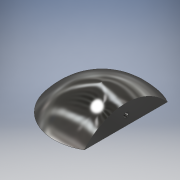
# Autodesk Inventor part: camera side 2
Saved by Autodesk Inventor 2017 (Build 210142000, 142)
## iProperties
Created: 2020-02-20
Part Number: camera side 2
Material: Silicon Nitride
Document SubType Name: Modeling
Designer: S346852600
Density: 3.18 g/cm^3
Appearance: Chrome - Polished Black
Author: S346852600
Autodesk Inventor part; units mm, degrees
ref_plane "YZ Plane" through (0, 0, 0) normal (1, 0, 0) x (0, 1, 0)
ref_plane "XZ Plane" through (0, 0, 0) normal (0, 1, 0) x (-1, 0, 0)
ref_plane "XY Plane" through (0, 0, 0) normal (0, 0, 1) x (1, 0, 0)
sketch "Sketch1" plane through (0, 0, 0) normal (1, 0, 0) x (0, 1, 0)
  line L0 (0, 0) -> (0, 25.4)
  line L1 (0, 0) -> (13.97, 0)
  arc A0 (13.97, 0) -> (0, 25.4) centre (-21.4675, -2.9489) ccw
  line L2 (0, 0) -> (0, 15.748)
  line L3 (0, 15.748) -> (8.7805, 15.748)
  dimension "d0" = 25.4
  dimension "d1" = 13.97
  dimension "d2" = 35.56
  dimension "d3" = 15.748
  constraints: 8 end point, 3 point on circle, 1 centre point, 1 horizontal, 1 perpendicular, 1 point on line, 1 vertical
  measures "d0" distance of L0.start L0.end
  measures "d1" distance of L0.start L1.end
  measures "d2" radius of A0
  measures "d3" distance of L0.start L2.end
revolve "Revolution1" add sketch "Sketch1" angle 360 about axis through (0, 0, 0) along (0, 1, 0)
sketch "Sketch6" plane through (0, 0, 0) normal (0, -1, 0) x (0, 0, -1)
  circle A0 centre (0, 0) radius 1.27
  dimension "d19" = 2.54
  constraints: 1 centre point, 1 coincident
  measures "d19" diameter of A0
extrude "Extrusion5" cut sketch "Sketch6" against normal blind 2.54
sketch "Sketch7" plane through (0, 0, 0) normal (0, -1, 0) x (0, 0, -1)
  point P0 (0, 0)
sketch "Sketch8" plane through (0, 0, 0) normal (0, -1, 0) x (1, 0, 0)
  circle A0 centre (0, 0) radius 1.27 projected
  line L0 (0, 0) -> (12.657, 0)
  line L1 (12.657, 0) -> (12.657, 22.0218)
  circle A1 centre (0, 0) radius 25.4 projected
  line L2 (12.657, 22.0218) -> (27.5297, 22.0218)
  line L3 (27.5297, 22.0218) -> (27.5297, -29.4448)
  line L4 (27.5297, -29.4448) -> (12.657, -29.4448)
  line L5 (12.657, -29.4448) -> (12.657, 22.0218)
  dimension "d22" = 22.0218
  constraints: 12 end point, 2 horizontal, 2 parallel, 2 perpendicular, 2 other
  measures "d22" distance of L0.end L1.end
extrude "Extrusion6" cut sketch "Sketch8" against normal blind 25.4 contours L1 A1 L5 | L2 L3 L4 L5 A1 picked at (14.0935, 13.6414)
sketch "Sketch9" plane through (12.657, 0, 22.0218) normal (1, 0, 0) x (0, 0, -1)
  line L0 (22.0218, 0) -> (22.0218, 5.08)
  circle A0 centre (22.0218, 5.08) radius 1.27
  dimension "d25" = 5.08
  dimension "d26" = 2.54
  constraints: 2 end point, 1 centre point, 1 coincident, 1 vertical
  measures "d25" distance of L0.start L0.end
  measures "d26" diameter of A0
extrude "Extrusion7" cut sketch "Sketch9" against normal blind 2.54
body "Solid1"
